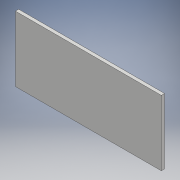
# Autodesk Inventor part: 盖板
Saved by Autodesk Inventor 2018 (Build 220112000, 112)
## iProperties
Created: 2020-11-30
Part Number: 盖板
Material: 常规
Document SubType Name: Modeling
Designer: OHHHHHHHHHH
Density: 1 g/cm^3
Appearance: 默认
Author: OHHHHHHHHHH
Autodesk Inventor part; units mm, degrees
ref_plane "YZ Plane" through (0, 0, 0) normal (1, 0, 0) x (0, 1, 0)
ref_plane "XZ Plane" through (0, 0, 0) normal (0, 1, 0) x (-1, 0, 0)
ref_plane "XY Plane" through (0, 0, 0) normal (0, 0, 1) x (1, 0, 0)
sketch "草图1" plane through (0, 0, 0) normal (0, 1, 0) x (-1, 0, 0)
  line L0 (0, 0) -> (67, 0)
  line L1 (67, 0) -> (67, -30)
  line L2 (67, -30) -> (0, -30)
  line L3 (0, -30) -> (0, 0)
  dimension "d0" = 30
  dimension "d3" = 67
  constraints: 8 end point, 2 parallel, 1 horizontal, 1 perpendicular
  measures "d0" distance of L0.end L1.end
  measures "d3" distance of L1.end L2.end
extrude "拉伸1" add sketch "草图1" along normal blind 1.5
